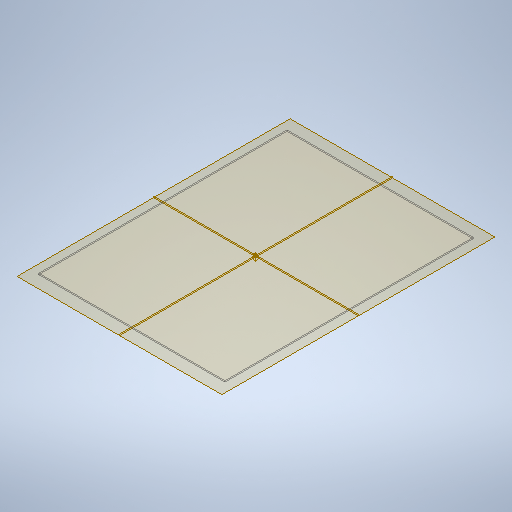
# Autodesk Inventor part: ground
Saved by Autodesk Inventor 2025.2 (Build 292293000, 293)
## iProperties
Created: 2025-03-23
Part Number: ground
Material: PET Plastic
Document SubType Name: Modeling
Designer: MSIGAMING
Mass: 15410 g
Surface Area: 20400 cm^2
Volume: 10000 cm^3
Density: 1.541 g/cm^3
Appearance: Polycarbonate - Clear
Author: MSIGAMING
Autodesk Inventor part; units mm, degrees
sketch "Sketch1" plane through (0, 0, 0) normal (0, 1, 0) x (-1, 0, 0)
  line L0 (-750, -1000) -> (750, -1000)
  line L1 (750, -1000) -> (750, 1000)
  line L2 (750, 1000) -> (-750, 1000)
  line L3 (-750, 1000) -> (-750, -1000)
  line L4 (-750, -1000) -> (750, 1000) construction
  line L5 (750, -1000) -> (-750, 1000) construction
  point P0 (0, 0)
  dimension "d0" = 1500
  dimension "d1" = 2000
  constraints: 12 end point, 2 midpoint, 2 parallel, 1 horizontal, 1 perpendicular
  measures "d0" distance of L2.end L1.end
  measures "d1" distance of L1.end L0.end
extrude "Extrusion1" add sketch "Sketch1" along normal blind 10
body "Solid1"
